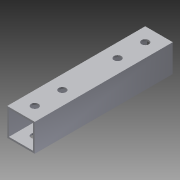
# Autodesk Inventor part: Square Tube 1-16 thick Support
Saved by Autodesk Inventor 2014 (Build 180170000, 170)
## iProperties
Created: 2014-02-10
Part Number: Square Tube 1-16 thick Support
Material: Aluminum 6061
Document SubType Name: Modeling
Designer: Michael
Density: 2.71 g/cm^3
Appearance: Aluminum - Flat
Author: Michael
Autodesk Inventor part; units mm, degrees
ref_plane "YZ Plane" through (0, 0, 0) normal (1, 0, 0) x (0, 1, 0)
ref_plane "XZ Plane" through (0, 0, 0) normal (0, 1, 0) x (-1, 0, 0)
ref_plane "XY Plane" through (0, 0, 0) normal (0, 0, 1) x (1, 0, 0)
sketch "Sketch1" plane through (0, 0, 0) normal (0, 0, 1) x (1, 0, 0)
  line L0 (0, 0) -> (25.4, 0)
  line L1 (25.4, 0) -> (25.4, 25.4)
  line L2 (25.4, 25.4) -> (0, 25.4)
  line L3 (0, 25.4) -> (0, 0)
  line L4 (1.5875, 23.8125) -> (23.8125, 23.8125)
  line L5 (23.8125, 23.8125) -> (23.8125, 1.5875)
  line L6 (23.8125, 1.5875) -> (1.5875, 1.5875)
  line L7 (1.5875, 1.5875) -> (1.5875, 23.8125)
  dimension "d0" = 25.4
  dimension "d1" = 25.4
  dimension "d2" = 1.5875
  constraints: 16 end point, 4 parallel, 2 perpendicular, 1 horizontal, 3 other
  measures "d0" distance of L2.end L1.end
  measures "d1" distance of L1.end L0.end
  measures "d2" distance between parallel lines of L2 L4
extrude "Extrusion1" add sketch "Sketch1" along normal blind 127
sketch "Sketch2" plane through (0, 25.4, 0) normal (0, 1, 0) x (1, 0, 0)
  line L0 (25.4, 0) -> (0, 0) projected
  line L1 (0, 0) -> (0, -127) projected
  line L2 (25.4, 0) -> (25.4, -127) projected
  circle A0 centre (12.7, -12.7) radius 3.3782
  circle A1 centre (12.7, -38.1) radius 3.3782
  circle A2 centre (12.7, -88.9) radius 3.3782
  circle A3 centre (12.7, -114.3) radius 3.3782
  dimension "d5" = 6.7564
  dimension "d6" = 12.7
  dimension "d7" = 12.7
  dimension "d10" = 25.4
  dimension "d17" = 12.7
  dimension "d18" = 50.8
  dimension "d21" = 25.4
  constraints: 4 centre point, 2 vertical, 1 equal radius, 4 other
  measures "d5" diameter of A0
  measures "d6" distance from line of L0 A0.centre
  measures "d7" distance from line of L2 A0.centre
  measures "d10" distance of A0.centre A1.centre
  measures "d17" distance from line of L1 A2.centre
  measures "d18" distance of A1.centre A2.centre
  measures "d21" distance of A2.centre A3.centre
extrude "Extrusion2" cut sketch "Sketch2" against normal blind 101.6
body "Solid1"
